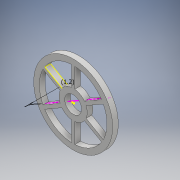
# Autodesk Inventor part: 앞바퀴
Saved by Autodesk Inventor 2018 (Build 220112000, 112)
## iProperties
Created: 2019-11-05
Part Number: 앞바퀴
Material: 일반
Document SubType Name: Modeling
Designer: LeeYounSeo
Density: 1 g/cm^3
Appearance: 기본값
Author: LeeYounSeo
Autodesk Inventor part; units mm, degrees
ref_plane "YZ Plane" through (0, 0, 0) normal (1, 0, 0) x (0, 1, 0)
ref_plane "XZ Plane" through (0, 0, 0) normal (0, 1, 0) x (-1, 0, 0)
ref_plane "XY Plane" through (0, 0, 0) normal (0, 0, 1) x (1, 0, 0)
sketch "스케치1" plane through (0, 0, 0) normal (0, 1, 0) x (-1, 0, 0)
  circle A0 centre (0, 0) radius 35
  circle A1 centre (0, 0) radius 7.5
  circle A2 centre (0, 0) radius 12.5
  circle A3 centre (0, 0) radius 30
  dimension "d0" = 70
  dimension "d1" = 15
  dimension "d2" = 25
  dimension "d3" = 60
  constraints: 4 centre point, 4 coincident
  measures "d0" diameter of A0
  measures "d1" diameter of A1
  measures "d2" diameter of A2
  measures "d3" diameter of A3
extrude "돌출1" add sketch "스케치1" along normal blind 5
sketch "스케치2" plane through (0, 0, 0) normal (0, -1, 0) x (1, 0, 0)
  line L0 (-10.8253, 6.25) -> (-25.9808, 15)
  circle A0 centre (0, 0) radius 30 projected
  circle A1 centre (0, 0) radius 7.5 projected
  circle A2 centre (0, 0) radius 7.5 projected
  circle A3 centre (0, 0) radius 12.5 projected
  circle A4 centre (0, 0) radius 12.5 projected
  line L1 (0, 12.5) -> (0, 30)
  line L2 (10.8253, 6.25) -> (25.9808, 15)
  line L3 (10.8253, -6.25) -> (25.9808, -15)
  line L4 (0, -12.5) -> (0, -30)
  line L5 (-10.8253, -6.25) -> (-25.9808, -15)
  line L6 (-1.5, 34.9678) -> (1.5, 34.9678)
  line L7 (1.5, 34.9678) -> (1.5, 12.4097)
  line L8 (1.5, 12.4097) -> (-1.5, 12.4097)
  line L9 (-1.5, 12.4097) -> (-1.5, 34.9678)
  circle A5 centre (0, 0) radius 35 projected
  dimension "d10" = 3
  dimension "d11" = 1.5
  constraints: 20 end point, 14 point on circle, 3 equal length, 1 horizontal, 1 perpendicular, 1 vertical alignment, 2 other
  measures "d10" distance between parallel lines of L7 L9
  measures "d11" distance between parallel lines of L1 L7
extrude "돌출2" add sketch "스케치2" against normal blind 5 contours L9 A0 L1 A3 | L9 L6 L7 A0 | L1 A0 L7 A3
pattern_circular "원형 패턴1" count 6 over 360 about axis through (0, 0, 0) along (0, 1, 0) of "돌출2"
sketch "스케치3" plane through (-26.6983, 0, -13.6822) normal (-0.5, 0, 0.866) x (0.866, 0, 0.5)
  line L0 (64.9625, 3.1) -> (-5.0375, 3.1) projected
  line L1 (-5.0375, 1.9) -> (64.9625, 1.9) projected
  point P0 (29.9625, 0)
  dimension "d18" = 1.2
  measures "d18" distance between parallel lines of L0 L1
sketch "스케치6" plane through (-25.1983, 0, 16.2803) normal (0.5, 0, 0.866) x (0.866, 0, -0.5)
  line L0 (0, 0) -> (0, 5) projected
  line L1 (17.5528, 0) -> (0, 0) projected
  line L2 (17.5528, 5) -> (17.5528, 0) projected
  line L3 (0, 5) -> (17.5528, 5) projected
  point P0 (29.9625, 0)
